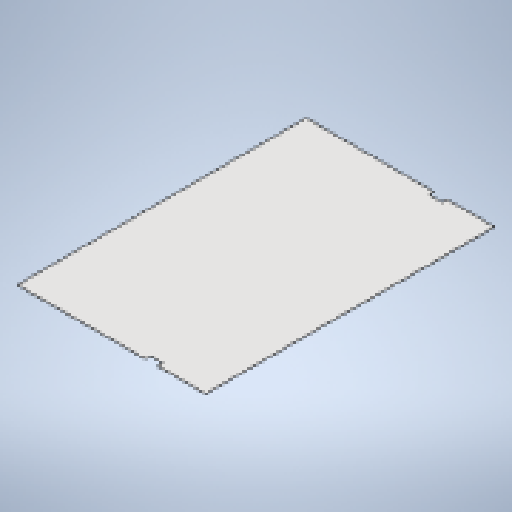
# Autodesk Inventor part: GnG L.2 floor sheet
Saved by Autodesk Inventor 2025 (Build 290162010, 162A)
## iProperties
Created: 2025-10-28
Part Number: GnG L.2 floor sheet
Material: Stainless Steel
Document SubType Name: Sheet Metal
Designer: admin
Mass: 280.619 g
Surface Area: 364.406 cm^2
Volume: 35.0774 cm^3
Density: 8 g/cm^3
Sheet Metal Rule: AISI304 3mm Die 32
Sheet Metal Width: 1500,000 mm
Sheet Metal Length: 2300,000 mm
Sheet Metal Area: 3450000,000 mm^2
Appearance: Default
Stock Number: L2
Flat Pattern Width: 150 cm
Flat Pattern Length: 230 cm
Flat Pattern Area: 34500 cm^2
Author: admin
Autodesk Inventor part; units mm, degrees
ref_plane "YZ Plane" through (0, 0, 0) normal (1, 0, 0) x (0, 1, 0)
ref_plane "XZ Plane" through (0, 0, 0) normal (0, 1, 0) x (-1, 0, 0)
ref_plane "XY Plane" through (0, 0, 0) normal (0, 0, 1) x (1, 0, 0)
sketch "Sketch1" plane through (0, 0, 0) normal (0, 0, 1) x (1, 0, 0)
  line L0 (0, 0) -> (-1500, 0)
  line L1 (-1500, 0) -> (-1500, -2300)
  line L2 (-1500, -2300) -> (0, -2300)
  line L3 (0, -2300) -> (0, 0)
  line L4 (0, 0) -> (-40, 0)
  line L5 (-40, 0) -> (-40, -40)
  line L6 (-40, -40) -> (0, -40)
  line L7 (0, -40) -> (0, 0)
  line L8 (0, -2300) -> (-40, -2300)
  line L9 (-40, -2300) -> (-40, -2260)
  line L10 (-40, -2260) -> (0, -2260)
  line L11 (0, -2260) -> (0, -2300)
  line L12 (-1500, 0) -> (-1460, 0)
  line L13 (-1460, 0) -> (-1460, -40)
  line L14 (-1460, -40) -> (-1500, -40)
  line L15 (-1500, -40) -> (-1500, 0)
  line L16 (-1500, -2300) -> (-1460, -2300)
  line L17 (-1460, -2300) -> (-1460, -2260)
  line L18 (-1460, -2260) -> (-1500, -2260)
  line L19 (-1500, -2260) -> (-1500, -2300)
  line L20 (-480, -2300) -> (-380, -2300)
  line L21 (-380, -2300) -> (-380, -2260)
  line L22 (-380, -2260) -> (-480, -2260)
  line L23 (-480, -2260) -> (-480, -2300)
  line L24 (-480, 0) -> (-380, 0)
  line L25 (-380, 0) -> (-380, -40)
  line L26 (-380, -40) -> (-480, -40)
  line L27 (-480, -40) -> (-480, 0)
  point P0 (0, -40)
  point P1 (-40, 0)
  point P2 (0, -2260)
  point P3 (-380, -2300)
  point P4 (-380, 0)
  dimension "d22" = 1500
  dimension "d23" = 2300
  dimension "d24" = 40
  dimension "d25" = 40
  dimension "d28" = 100
  dimension "d29" = 340
  measures "d22" distance of L2.end L1.end
  measures "d23" distance of L1.end L0.end
  measures "d24" distance of L6.end L5.end
  measures "d25" distance of L5.end L4.end
  measures "d28" distance of L25.end L26.end
  measures "d29" distance between parallel lines of L5 L25
extrude "Plate1" add sketch "Sketch1" along normal blind 3 contours L3 L6 L5 L0 | L5 L6 L3 L10 L9 L2 L21 L22 L23 L17 L18 L1 L14 L13 L0 L27 L26 L25 | L3 L2 L9 L10 | L13 L14 L1 L0 | L18 L17 L2 L1
sketch "Sketch6" plane through (0, 0, 3) normal (0, 0, 1) x (1, 0, 0)
  line L0 (0, 0) -> (0, -2300) projected
  line L1 (-380, 0) -> (0, 0) projected
  line L2 (-380, -40) -> (-380, 0) projected
  line L3 (-480, -40) -> (-380, -40) projected
  line L4 (-480, 0) -> (-480, -40) projected
  line L5 (-1500, 0) -> (-480, 0) projected
  line L6 (-1500, -2300) -> (-1500, 0) projected
  line L7 (-480, -2300) -> (-1500, -2300) projected
  line L8 (-480, -2260) -> (-480, -2300) projected
  line L9 (-380, -2260) -> (-480, -2260) projected
  line L10 (-380, -2300) -> (-380, -2260) projected
  line L11 (0, -2300) -> (-380, -2300) projected
  line L12 (-1395, 0) -> (-1390, 0)
  line L13 (-1390, 0) -> (-1390, -2)
  line L14 (-1390, -2) -> (-1395, -2)
  line L15 (-1395, -2) -> (-1395, 0)
  line L16 (-1375.2303, 0) -> (-1370.2303, 0)
  line L17 (-1370.2303, 0) -> (-1370.2303, -2)
  line L18 (-1370.2303, -2) -> (-1375.2303, -2)
  line L19 (-1375.2303, -2) -> (-1375.2303, 0)
  line L20 (-1385.2303, 0) -> (-1380.2303, 0)
  line L21 (-1380.2303, 0) -> (-1380.2303, -2)
  line L22 (-1380.2303, -2) -> (-1385.2303, -2)
  line L23 (-1385.2303, -2) -> (-1385.2303, 0)
  line L24 (-1365.2303, 0) -> (-1362.2303, 0)
  line L25 (-1380.2303, -1) -> (-1375.2303, -1)
  line L26 (-1365.2303, 0) -> (-1364.9363, -1.0787)
  arc A0 (-1364.9363, -1.0787) -> (-1362.5243, -1.0787) centre (-1363.7303, -0.75) ccw
  line L27 (-1362.5243, -1.0787) -> (-1362.2303, 0)
  line L28 (-1370.2303, 0) -> (-1365.2303, 0)
  line L29 (-1342.2303, -2) -> (-1347.2303, -2)
  line L30 (-1342.2303, -1) -> (-1337.2303, -1)
  line L31 (-1352.2303, -2) -> (-1357.2303, -2)
  line L32 (-1352.2303, -1) -> (-1347.2303, -1)
  line L33 (-1347.2303, 0) -> (-1342.2303, 0)
  line L34 (-1347.2303, -2) -> (-1347.2303, 0)
  line L35 (-1357.2303, 0) -> (-1352.2303, 0)
  line L36 (-1357.2303, -2) -> (-1357.2303, 0)
  line L37 (-1352.2303, 0) -> (-1352.2303, -2)
  line L38 (-1342.2303, 0) -> (-1342.2303, -2)
  line L39 (-1337.2303, -2) -> (-1337.2303, 0)
  line L40 (-1337.2303, 0) -> (-1332.2303, 0)
  line L41 (-1332.2303, 0) -> (-1332.2303, -2)
  line L42 (-1332.2303, -2) -> (-1337.2303, -2)
  line L43 (-1362.2303, 0) -> (-1357.2303, 0)
  circle A1 centre (-1400, 0) radius 2.5
  line L44 (-1500, 0) -> (-480, 0) projected
  point P0 (-1363.7303, 0)
  point P1 (-1397.5, 0)
  point P2 (-1402.5, 0)
  point P3 (-1390, 0)
  point P4 (-1395, 0)
  point P5 (-1380.2303, 0)
  point P6 (-1385.2303, 0)
  dimension "d38" = 5
  dimension "d39" = 2
  dimension "d40" = 1.25
  dimension "d41" = 3
  dimension "d42" = 5
  dimension "d44" = 5
  dimension "d45" = 5
  dimension "d46" = 100
  constraints: 64 end point, 12 parallel, 11 horizontal, 7 equal length, 7 midpoint, 6 collinear, 6 perpendicular, 3 tangent, 2 centre point, 2 point on circle, 2 point on line, 1 vertical alignment
  measures "d38" distance of L13.end L14.end
  measures "d39" distance of L14.end L12.start
  measures "d40" radius of A0
  measures "d41" distance of L28.end L24.end
  measures "d42" distance of L31.start L36.start
  measures "d44" diameter of A1
  measures "d45" distance of A1.centre L12.start
  measures "d46" distance from line of L6 A1.centre
extrude "Cut1" cut sketch "Sketch6" against normal blind 3 contours L5 A1 | L5 L13 L14 L15 | L5 L21 L22 L23 picked at (-1400.7379, -0.3873)
equation "\"d24\" = d25"
equation "\"d40\" = 0.25 * d38"
equation "\"d47\" = Thickness"
equation "\"d2\" = Thickness"
equation "\"BendReliefWidth\" = Thickness"
equation "\"BendReliefDepth\" = 0.5 * Thickness"
equation "\"CornerReliefSize\" = 4 * Thickness"
equation "\"MinimumRemnant\" = 2 * Thickness"
equation "\"TransitionRadius\" = BendRadius"
equation "\"JacobiRadiusSize\" = BendRadius"
equation "\"GapSize\" = Thickness"
equation "\"Thickness\" = 3"
equation "\"BendRadius\" = 5"
body "Solid1"
